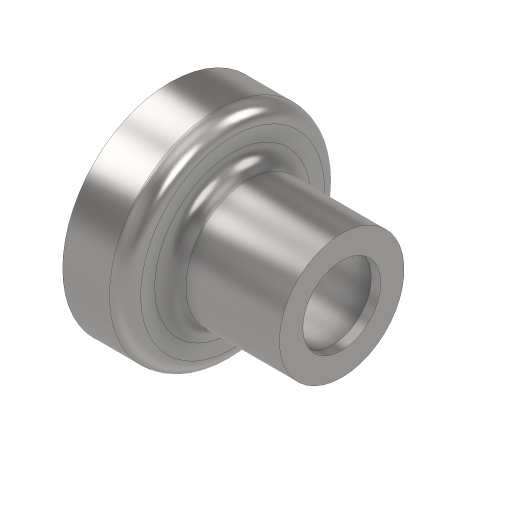
# Autodesk Inventor part: Part3
Saved by Autodesk Inventor 2024.2 (Build 282272000, 272)
## iProperties
Created: 2019-06-28
Part Number: Part3
Material: Stainless Steel
Document SubType Name: Modeling
Designer: Nakamura
Density: 8 g/cm^3
Appearance: Semi-Polished
Mass: 2.7973 g
Surface Area: 6.70416 cm^2
Volume: 0.349662 cm^3
Author: Nakamura
Autodesk Inventor part; units mm, degrees
ref_plane "YZ Plane" through (0, 0, 0) normal (1, 0, 0) x (0, 1, 0)
ref_plane "XZ Plane" through (0, 0, 0) normal (0, 1, 0) x (-1, 0, 0)
ref_plane "XY Plane" through (0, 0, 0) normal (0, 0, 1) x (1, 0, 0)
sketch "スケッチ1" plane through (0, 0, 0) normal (0, 0, 1) x (1, 0, 0)
  line L0 (0, 0) -> (11, 0)
  line L1 (11, 0) -> (11, 4)
  line L2 (11, 4) -> (4, 4)
  line L3 (4, 4) -> (4, 6.9)
  line L4 (4, 6.9) -> (0, 6.9)
  line L5 (0, 6.9) -> (0, 0)
  dimension "d9" = 8
  dimension "d10" = 13.8
  dimension "d11" = 4
  dimension "d12" = 7
  constraints: 12 end point, 4 perpendicular, 1 horizontal, 1 vertical
  measures "d9" diameter of L2 L0
  measures "d10" diameter of L4 L0
  measures "d11" distance of L3.end L4.end
  measures "d12" distance of L1.end L2.end
revolve "回転1" add sketch "スケッチ1" angle 360 about axis through (0, 0, 0) along (1, 0, 0)
shell "Shell1" thickness 0.6 removed faces 1 at (0, 1.1832, -1.6579)
sketch "Sketch2" plane through (11, 0, 0) normal (1, 0, 0) x (0, 0, -1)
  circle A0 centre (0, 0) radius 2.5
  dimension "d14" = 5
  constraints: 1 centre point, 1 coincident
  measures "d14" diameter of A0
extrude "Extrusion1" cut sketch "Sketch2" against normal blind 11
fillet "Fillet1" radius 1 2 edges at (4, -6.9, 0) (4, -4, 0)
